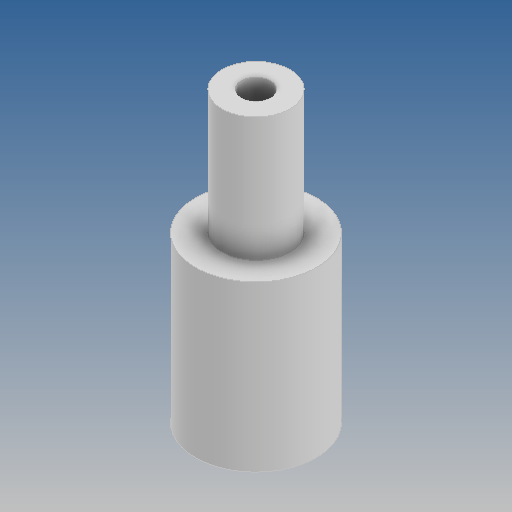
# Autodesk Inventor part: 0008-30-1008 Adaptor furtun
Saved by Autodesk Inventor 2020 (Build 240168000, 168)
## iProperties
Created: 2021-06-01
Part Number: 0008-30-1008 Adaptor furtun
Material: Generic
Document SubType Name: Modeling
Designer: Iulian Bors
Density: 1 g/cm^3
Appearance: Default
Author: Iulian Bors
Subject: 1008
Autodesk Inventor part; units mm, degrees
ref_plane "YZ Plane" through (0, 0, 0) normal (1, 0, 0) x (0, 1, 0)
ref_plane "XZ Plane" through (0, 0, 0) normal (0, 1, 0) x (-1, 0, 0)
ref_plane "XY Plane" through (0, 0, 0) normal (0, 0, 1) x (1, 0, 0)
sketch "Sketch1" plane through (0, 0, 0) normal (0, 0, 1) x (1, 0, 0)
  line L0 (0, 2.4022) -> (0, -2.2164) construction
  line L1 (-3.35, 13.4) -> (-3.35, 0)
  line L2 (-4.92, 13.4) -> (-4.92, 0)
  line L3 (-4.92, 13.4) -> (-3.35, 13.4)
  line L4 (-4.92, 11.83) -> (-1.2, 11.83)
  line L5 (-1.2, 11.83) -> (-1.2, 23.5)
  line L6 (-3.35, 13.4) -> (-1.2, 13.4)
  line L7 (-2.77, 13.4) -> (-2.77, 23.5)
  line L8 (-4.92, 0) -> (-3.35, 0)
  line L9 (-2.77, 23.5) -> (-1.2, 23.5)
  point P0 (0, 0)
  point P1 (0, 0.0929)
  point P2 (-3.35, 11.83)
  dimension "d0" = 3.35
  dimension "d1" = 13.4
  dimension "d2" = 1.57
  dimension "d3" = 1.57
  dimension "d4" = 1.2
  dimension "d5" = 1.57
  dimension "d7" = 23.5
  constraints: 20 end point, 5 vertical, 4 horizontal, 4 horizontal alignment, 3 point on line, 1 midpoint, 1 parallel, 1 perpendicular, 1 vertical alignment
  measures "d0" distance between parallel lines of L0 L1
  measures "d1" distance of L1.start L1.end
  measures "d2" distance between parallel lines of L1 L2
  measures "d3" distance between parallel lines of L3 L4
  measures "d4" distance between parallel lines of L0 L5
  measures "d5" distance between parallel lines of L5 L7
  measures "d7" vertical distance of L1.end L5.end
revolve "Revolution1" add sketch "Sketch1" angle 360 about axis through (0, 2.4022, 0) along (0, -1, 0)
equation "\"d3\" = d2"
equation "\"d5\" = d2"
body "Solid1"
